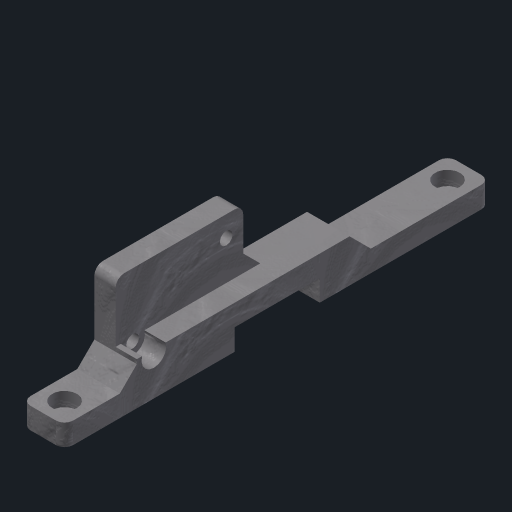
# Autodesk Inventor part: SOPORTE_FIN_CARRERA_INGRESO
Saved by Autodesk Inventor 2024.3 (Build 283343000, 343)
## iProperties
Created: 2024-07-21
Part Number: SOPORTE_FIN_CARRERA_INGRESO
Material: Steel, Mild, Welded
Document SubType Name: Modeling
Designer: Niler
Density: 7.85 g/cm^3
Appearance: Weld - Steel Mild
Author: Niler
Autodesk Inventor part; units mm, degrees
ref_plane "YZ Plane" through (0, 0, 0) normal (1, 0, 0) x (0, 1, 0)
ref_plane "XZ Plane" through (0, 0, 0) normal (0, 1, 0) x (-1, 0, 0)
ref_plane "XY Plane" through (0, 0, 0) normal (0, 0, 1) x (1, 0, 0)
sketch "Sketch1" plane through (0, 0, 0) normal (0, 1, 0) x (-1, 0, 0)
  line L0 (-5, 50) -> (5, 50)
  line L1 (5, 50) -> (5, -50)
  line L2 (5, -50) -> (-5, -50)
  line L3 (-5, -50) -> (-5, 50)
  line L4 (-5, 50) -> (5, -50) construction
  line L5 (5, 50) -> (-5, -50) construction
  circle A0 centre (0, 45) radius 1.65
  circle A1 centre (0, -45) radius 1.65
  line L6 (0, 45) -> (0, -45) construction
  line L7 (-5, -10) -> (5, -10)
  line L8 (5, -10) -> (5, 10)
  line L9 (5, 10) -> (-5, 10)
  line L10 (-5, 10) -> (-5, -10)
  line L11 (-5, -10) -> (5, 10) construction
  line L12 (5, -10) -> (-5, 10) construction
  point P0 (0, 0)
  dimension "d0" = 90
  dimension "d1" = 5
  dimension "d2" = 3.3
  dimension "d3" = 10
  dimension "d4" = 20
  constraints: 26 end point, 5 midpoint, 4 parallel, 2 centre point, 2 horizontal, 2 perpendicular, 1 equal radius, 1 point on line, 1 vertical, 1 vertical alignment
  measures "d0" distance of L6.start L6.end
  measures "d1" distance from line of L0 L6.start
  measures "d2" diameter of A0
  measures "d3" distance of L0.start L0.end
  measures "d4" distance between parallel lines of L7 L9
extrude "Extrusion1" add sketch "Sketch1" along normal blind 5 contours L0 L1 L9 L3 | L7 L1 L2 L3
sketch "Sketch2" plane through (0, 5, 0) normal (0, 1, 0) x (1, 0, 0)
  line L0 (5, -50) -> (5, -10) projected
  line L1 (5, -10) -> (-5, -10) projected
  line L2 (-5, -10) -> (-5, -50) projected
  line L3 (-5, -50) -> (5, -50) projected
  circle A0 centre (0, -45) radius 1.65 projected
  line L4 (-5, 50) -> (-5, 10) projected
  line L5 (-5, 10) -> (5, 10) projected
  line L6 (5, 10) -> (5, 50) projected
  line L7 (5, 50) -> (-5, 50) projected
  circle A1 centre (0, 45) radius 1.65 projected
  line L8 (-5, -33) -> (5, -33)
  line L9 (5, -33) -> (5, 17)
  line L10 (5, 17) -> (-5, 17)
  line L11 (-5, 17) -> (-5, -33)
  point P0 (0, 0)
  point P1 (5, -33)
  point P2 (-5, 17)
  dimension "d7" = 50
  dimension "d26" = 7
  constraints: 8 end point, 2 parallel, 2 point on line, 1 horizontal, 1 perpendicular
  measures "d7" distance of L8.end L9.end
  measures "d26" distance between parallel lines of L10 L5
extrude "Extrusion2" add sketch "Sketch2" along normal blind 5 contours L8 L2 L1 L0 | L1 L11 L5 L9 | L5 L4 L10 L6
sketch "Sketch3" plane through (0, 10, 0) normal (0, 1, 0) x (1, 0, 0)
  line L0 (5, -33) -> (5, 17) projected
  line L1 (5, 17) -> (-5, 17) projected
  line L2 (-5, 17) -> (-5, -33) projected
  line L3 (-5, -33) -> (5, -33) projected
  line L4 (-5, -3) -> (0, -3)
  line L5 (0, -3) -> (0, -33)
  line L6 (0, -33) -> (-5, -33)
  line L7 (-5, -33) -> (-5, -3)
  point P0 (0, 0)
  point P1 (-5, -33)
  point P2 (0, -33)
  dimension "d10" = 5
  dimension "d11" = 30
  constraints: 8 end point, 2 parallel, 2 point on line, 1 horizontal, 1 midpoint, 1 perpendicular
  measures "d10" distance of L4.start L4.end
  measures "d11" distance of L4.end L5.end
extrude "Extrusion3" add sketch "Sketch3" along normal blind 14 contours L3 L2 L4 L5
sketch "Sketch4" plane through (-5, 0, -50) normal (-1, 0, 0) x (0, 0, 1)
  line L0 (0, 0) -> (40, 0) projected
  line L1 (40, 0) -> (40, 5) projected
  line L2 (40, 5) -> (60, 5) projected
  line L3 (60, 0) -> (60, 5) projected
  line L4 (60, 0) -> (100, 0) projected
  line L5 (100, 0) -> (100, 5) projected
  line L6 (83, 5) -> (100, 5) projected
  line L7 (83, 5) -> (83, 24) projected
  line L8 (33, 10) -> (53, 10) projected
  line L9 (53, 24) -> (83, 24) projected
  line L10 (53, 10) -> (53, 24) projected
  line L11 (33, 5) -> (33, 10) projected
  line L12 (0, 5) -> (33, 5) projected
  line L13 (0, 0) -> (0, 5) projected
  line L14 (54, 6.1345) -> (82, 6.1345)
  line L15 (82, 6.1345) -> (82, 22.1345)
  line L16 (82, 22.1345) -> (54, 22.1345)
  line L17 (54, 22.1345) -> (54, 6.1345)
  circle A0 centre (57, 19.1345) radius 1.5
  circle A1 centre (79, 9.1345) radius 1.5
  line L18 (82, 6.1345) -> (79, 6.1345) construction
  line L19 (79, 6.1345) -> (79, 9.1345) construction
  line L20 (79, 9.1345) -> (82, 9.1345) construction
  line L21 (82, 9.1345) -> (82, 6.1345) construction
  line L22 (54, 22.1345) -> (57, 22.1345) construction
  line L23 (57, 22.1345) -> (57, 19.1345) construction
  line L24 (57, 19.1345) -> (54, 19.1345) construction
  line L25 (54, 19.1345) -> (54, 22.1345) construction
  point P0 (50, 0)
  point P1 (68, 22.1345)
  point P2 (68, 24)
  dimension "d14" = 28
  dimension "d15" = 16
  dimension "d18" = 3
  dimension "d19" = 3
  dimension "d22" = 3
  dimension "d23" = 3
  dimension "d24" = 3
  dimension "d25" = 3
  constraints: 24 end point, 6 parallel, 3 horizontal, 3 perpendicular, 2 centre point, 2 coincident, 2 midpoint, 1 vertical alignment
  measures "d14" distance of L16.end L15.end
  measures "d15" distance of L15.end L14.end
  measures "d18" diameter of A0
  measures "d19" diameter of A1
  measures "d22" distance of L19.end L20.end
  measures "d23" distance of L18.end L19.end
  measures "d24" distance of L23.end L24.end
  measures "d25" distance of L22.end L23.end
extrude "Extrusion4" cut sketch "Sketch4" against normal through all contours A0 | A1
sketch "Sketch5" plane through (0, 5, 0) normal (0, 1, 0) x (1, 0, 0)
  circle A0 centre (0, 45) radius 1.65 projected
  line L0 (5, -33) -> (-5, -33) projected
  line L1 (-5, -33) -> (-5, -50) projected
  line L2 (-5, -50) -> (5, -50) projected
  line L3 (5, -50) -> (5, -33) projected
  circle A1 centre (0, -45) radius 1.65 projected
  line L4 (-5, 17) -> (5, 17) projected
  line L5 (5, 17) -> (5, 50) projected
  line L6 (5, 50) -> (-5, 50) projected
  line L7 (-5, 50) -> (-5, 17) projected
  circle A2 centre (0, 45) radius 1.65 projected
  circle A3 centre (0, 45) radius 2.9
  circle A4 centre (0, -45) radius 2.9
  point P0 (0, 0)
  dimension "d27" = 5.8
  dimension "d28" = 5.8
  constraints: 2 centre point, 2 coincident
  measures "d27" diameter of A3
  measures "d28" diameter of A4
extrude "Extrusion5" cut sketch "Sketch5" against normal blind 3.3 contours A0 | A1 | A3 | A4
chamfer "Chamfer1" distance 4 angle 45 2 edges at (0, 5, 33) (-2.5, 10, 3)
fillet "Fillet1" radius 2 2 edges at (-2.5, 24, 33) (-2.5, 24, 3)
sketch "Sketch6" plane through (5, 0, 50) normal (1, 0, 0) x (0, 0, -1)
  arc A0 (19.7749, 10) -> (22.2251, 10) centre (21, 9.1345) ccw projected
  line L0 (17, 10) -> (19.7749, 10) projected
  line L1 (17, 9) -> (17, 10) projected
  line L2 (13, 5) -> (17, 9) projected
  line L3 (0, 5) -> (13, 5) projected
  line L4 (0, 0) -> (0, 5) projected
  line L5 (0, 0) -> (40, 0) projected
  line L6 (40, 0) -> (40, 5) projected
  line L7 (40, 5) -> (60, 5) projected
  line L8 (60, 0) -> (60, 5) projected
  line L9 (60, 0) -> (100, 0) projected
  line L10 (100, 0) -> (100, 5) projected
  line L11 (67, 5) -> (100, 5) projected
  line L12 (67, 5) -> (67, 10) projected
  line L13 (22.2251, 10) -> (67, 10) projected
  circle A1 centre (21, 9.1345) radius 2.9
  point P0 (50, 0)
  dimension "d35" = 5.8
  constraints: 1 centre point, 1 coincident
  measures "d35" diameter of A1
extrude "Extrusion6" cut sketch "Sketch6" against normal up to surface (5 mm away) contours L0 A1 L13 A0 | A0 L13 A1 L0
chamfer "Chamfer2" distance 5 angle 45 1 edges at (0, 5, -17)
fillet "Fillet2" radius 2 4 edges at (-5, 2.5, 50) (5, 2.5, 50) (-5, 2.5, -50) (5, 2.5, -50)
body "Solid1"
